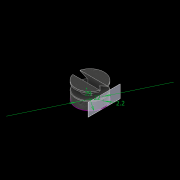
# Autodesk Inventor part: Part3
Saved by Autodesk Inventor 2019 (Build 230136000, 136)
## iProperties
Created: 2019-04-15
Part Number: Part3
Material: ABS Plastic
Document SubType Name: Modeling
Designer: skylercleland
Density: 1.06 g/cm^3
Appearance: Fine Textured - Black
Mass: 4.91222 g
Surface Area: 38.5812 cm^2
Volume: 4.63417 cm^3
Name: Ratchet
Author: skylercleland
Autodesk Inventor part; units mm, degrees
ref_plane "XZ Plane" through (0, 0, 0) normal (0, 1, 0) x (-1, 0, 0)
ref_plane "XY Plane" through (0, 0, 0) normal (0, 0, 1) x (1, 0, 0)
sketch "Sketch1" plane through (0, 0, 0) normal (0, 1, 0) x (-1, 0, 0)
  circle A0 centre (0, 0) radius 11
  circle A1 centre (0, 0) radius 14.5
  circle A2 centre (0, 0) radius 8.8
  dimension "d0" = 22
  dimension "d1" = 29
  dimension "d3" = 2.2
  constraints: 3 centre point, 3 coincident
  measures "d0" diameter of A0
  measures "d1" diameter of A1
  measures "d3" radial gap between concentric circles of A0 A2
extrude "Extrusion1" add sketch "Sketch1" along normal blind 16.9 contours A0 | A1 | A2
extrude "Extrusion2" cut sketch "Sketch1" along normal blind 7 contours A0 | A2
extrude "Extrusion3" cut sketch "Sketch1" along normal blind 7.1 contours A2
ref_plane "Work Plane1" through (14.5, 0, 0) normal (1, 0, 0) x (0, 1, 0)
sketch "Sketch2" plane through (14.5, 0, 0) normal (1, 0, 0) x (0, 1, 0)
  line L0 (7, -11) -> (7, 11) construction
  line L1 (7.1, -8.8) -> (7.1, 8.8) construction
  line L2 (8.5, 3.75) -> (16.9, 3.75)
  line L3 (16.9, 3.75) -> (16.9, -3.75)
  line L4 (16.9, -3.75) -> (8.5, -3.75)
  line L5 (8.5, -3.75) -> (8.5, 3.75)
  line L6 (8.5, 3.75) -> (16.9, -3.75) construction
  line L7 (16.9, 3.75) -> (8.5, -3.75) construction
  line L8 (16.9, -14.5) -> (16.9, 14.5) projected
  point P0 (0, 0)
  point P1 (12.7, 0)
  point P2 (12.7, 0)
  dimension "d11" = 7.5
  dimension "d27" = 1.5
  constraints: 12 end point, 3 midpoint, 2 parallel, 1 horizontal, 1 horizontal alignment, 1 perpendicular, 1 point on line
  measures "d11" distance between parallel lines of L4 L2
  measures "d27" distance between parallel lines of L0 L5
extrude "Extrusion4" cut sketch "Sketch2" against normal through all
sketch "Sketch5" plane through (0, 0, 0) normal (1, 0, 0) x (0, 1, 0)
  line L0 (8.5, 3.75) -> (8.5, -3.75) projected
  line L1 (8.5, -3.75) -> (16.9, -3.75) projected
  line L2 (16.9, 3.75) -> (8.5, 3.75) projected
  line L3 (16.9, -3.75) -> (8.5, -3.75) projected
  line L4 (8.5, -3.75) -> (8.5, 3.75) projected
  line L5 (8.5, 3.75) -> (16.9, 3.75) projected
  line L6 (16.9, -3.75) -> (16.9, -3.75) projected
  line L7 (0, -14.5) -> (16.9, -14.5) projected
  line L8 (15.5, -14.5) -> (8.5, -14.5)
  line L9 (8.5, -14.5) -> (8.5, -7.75)
  line L10 (8.5, -7.75) -> (12, -7.75)
  line L11 (12, -7.75) -> (15.5, -14.5)
  line L12 (-2.8, 0) -> (16.8, 0) projected
  line L13 (16.9, 3.75) -> (16.9, 3.75) projected
  point P0 (0, 0)
  point P1 (3, -15)
  point P2 (3, 15)
  point P3 (14, -14.5)
  point P4 (14, 14.5)
  dimension "d20" = 4
  dimension "d28" = 3.5
  dimension "d29" = 7
  constraints: 8 end point, 1 horizontal, 1 parallel, 1 perpendicular, 1 vertical alignment, 2 other
  measures "d20" distance between parallel lines of L1 L10
  measures "d28" distance of L9.end L10.end
  measures "d29" distance of L8.start L8.end
revolve "Revolution1" cut sketch "Sketch5" angle 360 about axis through (0, -10, 0) along (0, 1, 0)
fillet "Fillet1" radius 0.5 5 edges at (14.5, 8.5, 0) (6.7823, 10.25, 3.75) (6.7823, 10.25, -3.75) (-6.7823, 10.25, 3.75) (-6.7823, 10.25, -3.75)
fillet "Fillet2" radius 1 8 edges at (6.3297, 11.7963, -3.75) (9.8313, 13.4375, -3.75) (-6.3297, 11.7963, -3.75) (-9.8313, 13.4375, -3.75) (-6.3297, 11.7963, 3.75) (-9.8313, 13.4375, 3.75) (6.3297, 11.7963, 3.75) (9.8313, 13.4375, 3.75)
body "Solid1"
